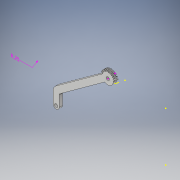
# Autodesk Inventor part: Beta_indexpt2
Saved by Autodesk Inventor 2018 (Build 220112000, 112)
## iProperties
Created: 2017-10-02
Part Number: Beta_indexpt2
Material: Generic
Document SubType Name: Modeling
Designer: rheal
Density: 1 g/cm^3
Appearance: Default
Author: rheal
Autodesk Inventor part; units mm, degrees
note: some values were not read from the file. Chosen so that the rebuilt part matches the saved one: pattern direction of "Circular Pattern2".
ref_plane "YZ Plane" through (0, 0, 0) normal (1, 0, 0) x (0, 1, 0)
ref_plane "XZ Plane" through (0, 0, 0) normal (0, 1, 0) x (-1, 0, 0)
ref_plane "XY Plane" through (0, 0, 0) normal (0, 0, 1) x (1, 0, 0)
sketch "Sketch1" plane through (0, 0, 0) normal (0, 0, 1) x (1, 0, 0)
  arc A0 (-100, 0) -> (-94.4595, -0.3204) centre (-97.2205, 0) ccw
  line L0 (-50, 32.0871) -> (-50, 50) construction
  arc A1 (-46.9563, 41.0331) -> (-50, 50) centre (-50, 45) ccw
  arc A2 (-52.8648, 40.9021) -> (-54.8116, 46.3594) centre (-50, 45) ccw
  line L1 (-100, 0) -> (-100, 10.4545)
  arc A3 (-100, 0) -> (-94.441, 0) centre (-97.2205, 0) ccw
  line L2 (-94.441, 0) -> (-94.441, 9.6967)
  line L3 (-93.616, 11.3151) -> (-52.8648, 40.9021)
  line L4 (-96.0743, 12.9658) -> (-97.7076, 15.2154)
  line L5 (-97.7076, 15.2154) -> (-54.8116, 46.3594)
  arc A4 (-97.7076, 15.2154) -> (-100, 10.4545) centre (-93.9101, 10.4545) ccw
  arc A5 (-93.616, 11.3151) -> (-94.441, 9.6967) centre (-92.441, 9.6967) ccw
  point P0 (19.05, 139.7)
  point P1 (-45.0077, 44.7222)
  point P2 (-94.441, 10.7162)
  dimension "d69" = 2.7795
  dimension "d100" = 2.78
  dimension "d103" = 2
  constraints: 14 point on circle, 12 end point, 6 centre point, 4 tangent, 2 point on line, 2 vertical, 1 coincident, 1 parallel
  measures "d69" radius of A0
  measures "d100" distance of point (-94.441, 10.716) L4.start
  measures "d103" radius of A5
extrude "Extrusion1" add sketch "Sketch1" along normal blind 3
sketch "Sketch12" plane through (0, 0, 3) normal (0, 0, 1) x (1, 0, 0)
  circle A0 centre (0, 0) radius 2.5
  arc A1 (-100, 0) -> (-94.4595, -0.3204) centre (-97.2205, 0) ccw projected
  circle A2 centre (-97.2205, 0) radius 1.5
  dimension "d70" = 5
  dimension "d71" = 3
  constraints: 2 centre point, 2 coincident
  measures "d70" diameter of A0
  measures "d71" diameter of A2
extrude "Extrusion11" cut sketch "Sketch12" against normal blind 5
sketch "Sketch13" plane through (-46.9563, 41.0331, 0) normal (0.608736, -0.7933729, 0) x (0.7933729, 0.608736, 0)
  line L0 (0, 0) -> (5, 0) projected
  point P0 (12.2755, 0)
sketch "Sketch15" plane through (0, 0, 0) normal (0, 0, -1) x (-1, 0, 0)
  point P0 (0, 0)
sketch "Sketch16" plane through (0, 0, 0) normal (0, 0, -1) x (-1, 0, 0)
  circle A0 centre (50, 45) radius 2.5 projected
  line L0 (50, 45) -> (50, 42.5) construction
  line L1 (50, 45) -> (52.5, 45) construction
  point P0 (0, 0)
  constraints: 4 end point, 2 point on circle, 1 perpendicular, 1 vertical
ref_plane "Work Plane2" through (-50, 45, 0) normal (0, -1, 0) x (1, 0, 0)
sketch "Sketch18" plane through (-50, 45, 0) normal (0, -1, 0) x (1, 0, 0)
  line L0 (0, 0.0908) -> (0, 2.9092) construction
  line L1 (0, 1.5) -> (0, -3.9375) construction
  point P0 (50, 0)
  constraints: 2 end point, 1 midpoint, 1 vertical
sketch "Sketch19" plane through (0, 0, 0) normal (0, 0, -1) x (-1, 0, 0)
  line L0 (40.2723, 49.5) -> (50, 49.5) construction
  line L1 (49.9882, 50.2217) -> (49.9882, 51.5) construction
  line L2 (49.9882, 49.7517) -> (49.4882, 49.7517)
  line L3 (49.7382, 51.5) -> (49.7382, 50.7199)
  arc A0 (49.7382, 50.7199) -> (49.4882, 49.7517) centre (51.3699, 49.7822) ccw
  line L4 (49.7382, 51.5) -> (49.9882, 51.5)
  line L5 (59.7277, 49.5) -> (50, 49.5) construction
  line L6 (49.9882, 49.7517) -> (50.4882, 49.7517)
  line L7 (50.2382, 51.5) -> (50.2382, 50.7199)
  arc A1 (50.4882, 49.7517) -> (50.2382, 50.7199) centre (48.6065, 49.7822) ccw
  line L8 (50.2382, 51.5) -> (49.9882, 51.5)
  point P0 (0, 0)
  point P1 (50, 50)
  dimension "d82" = 1.5
  dimension "d83" = 0.5
  dimension "d84" = 0.25
  dimension "d85" = 1
  dimension "d86" = 0.2486
  constraints: 18 end point, 4 point on circle, 4 symmetric about line, 2 centre point, 1 perpendicular, 1 vertical, 1 other
  measures "d82" distance of point (50, 50) L1.end
  measures "d83" distance of L2.start L2.end
  measures "d84" distance between parallel lines of L1 L3
  measures "d85" distance of L3.end L2.end
  measures "d86" distance of point (50, 50) L2.start
extrude "Extrusion13" add sketch "Sketch19" against normal blind 3
sketch "Sketch20" plane through (0, 0, 0) normal (0, 0, -1) x (-1, 0, 0)
  line L0 (45.7576, 49.2502) -> (46.1486, 48.8898) projected
  line L1 (46.9253, 49.5288) -> (46.647, 49.982) projected
  point P0 (0, 0)
sketch "Sketch21" plane through (0, 0, 0) normal (0, 0, -1) x (-1, 0, 0)
  arc A0 (49.5542, 49.9801) -> (46.9563, 41.0331) centre (50, 45) ccw projected
  circle A1 centre (50, 45) radius 1.5
  point P0 (0, 0)
  dimension "d94" = 3
  constraints: 1 centre point, 1 coincident
  measures "d94" diameter of A1
extrude "Extrusion15" cut sketch "Sketch21" against normal blind 3
pattern_circular "Circular Pattern2" count 10 over 142 about axis through (-50, 45, 0) along (0, 0, -1) of "Extrusion13" both ways yes
body "Solid1"
